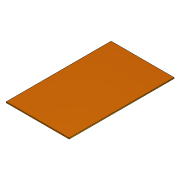
# Autodesk Inventor part: kapton_battery_tab
Saved by Autodesk Inventor 2014 SP1 (Build 180222100, 222)
## iProperties
Created: 2013-03-30
Part Number: kapton_battery_tab
Material: Acetal Resin, Black
Document SubType Name: Modeling
Designer: Robert Davis
Mass: 0.00855 g
Surface Area: 1.232 cm^2
Volume: 0.006 cm^3
Density: 1.425 g/cm^3
Appearance: Smooth - Medium Gray
Author: Robert Davis
Autodesk Inventor part; units mm, degrees
ref_plane "YZ Plane" through (0, 0, 0) normal (1, 0, 0) x (0, 1, 0)
ref_plane "XZ Plane" through (0, 0, 0) normal (0, 1, 0) x (-1, 0, 0)
ref_plane "XY Plane" through (0, 0, 0) normal (0, 0, 1) x (1, 0, 0)
sketch "Sketch1" plane through (0, 0, 0) normal (0, 0, 1) x (1, 0, 0)
  line L0 (0, 10.1631) -> (0, 0)
  line L1 (0, 0) -> (10.031, 0)
  line L2 (-3, 5) -> (3, 5)
  line L3 (3, 5) -> (3, -5)
  line L4 (3, -5) -> (-3, -5)
  line L5 (-3, -5) -> (-3, 5)
  dimension "d0" = 10
  dimension "d1" = 6
  constraints: 12 end point, 2 horizontal, 1 coincident, 1 vertical, 2 other
  measures "d0" distance of L2.end L3.end
  measures "d1" distance of L2.start L2.end
extrude "Extrusion1" add sketch "Sketch1" along normal blind 0.1
body "Solid1"
